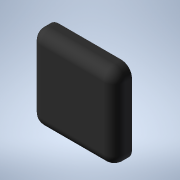
# Autodesk Inventor part: 0000-00189079(1)
Saved by Autodesk Inventor 2021 (Build 250183000, 183)
## iProperties
Created: 2025-05-05
Part Number: 0000-00189079(1)
Material: Generic
Catalog Web Link: www.cadenas.de
Description: Cap KL 2.0-Cap KL 2.0
Vendor: RITTAL
Document SubType Name: Modeling
Designer: psAdmin
Manufacturer: RITTAL
Mass: 0.993857 g
Surface Area: 6.97168 cm^2
Volume: 0.993857 cm^3
Density: 1 g/cm^3
Appearance: PSOLRGB-175-175-175
Category: PARTsolutions
Company: RITTAL
Title: 0000-00189079(1)
Author: Cadenas PARTsolutions
Comments: Cap KL 2.0
PSOL_IDENT_0: {$CADENAS_DATA/23d-libs/rittal/schaltschranksys/kleingeh/parts_kl_2_0/cap_kl_2_0.prj},188 {VTYP=3D},
PSOL_IDENT_1: {NB=0000-00189079(1)},{LINA=0000-00189079(1)},{NN=Cap KL 2.0},{DATE=27.11.2019 12:11:25},{GEOMDATE=2
PSOL_IDENT_2: 9.08.2019 12:58:38},{VERSION=},{LINEID=10},{WBVAR=DETAIL},{WBNUMERIC=DETAIL}  {NB=0000-00189079(1)},
PSOL_IDENT_3: {LINA=0000-00189079(1)},{KT=DUMMY},{BEST=0000-00189079},{DETAIL=1}
NB: 0000-00189079(1)
NN: Cap KL 2.0
NT: Cap KL 2.0
NBSYN: $BEST.($DETAIL.)
LINA: 0000-00189079(1)
CATALOG: Rittal
BEST: 0000-00189079
DETAIL: hoch
SUPPLIER: RITTAL
ARTICLENO: 0000-00189079(1)
BOMINFO: 0000-00189079(1)
CREATOR: CADENAS GmbH
Autodesk Inventor part; units mm, degrees
sketch "Sketch_4" plane through (0, 0, 0) normal (0, 1, 0) x (-1, 0, 0)
  arc A0 (7.75, -2) -> (5.75, 0) centre (5.75, -2) ccw
  line L0 (5.75, 0) -> (-5.75, 0)
  arc A1 (-5.75, 0) -> (-7.75, -2) centre (-5.75, -2) ccw
  line L1 (-7.75, -2) -> (-7.75, -3.25)
  line L2 (-7.75, -3.25) -> (7.75, -3.25)
  line L3 (7.75, -3.25) -> (7.75, -2)
  constraints: 8 end point, 4 point on circle, 2 centre point
extrude "Extrusion1" add sketch "Sketch_4" along normal mid plane 11.5
sketch "Sketch_5" plane through (0, 0, 0) normal (1, 0, 0) x (0, 1, 0)
  line L0 (5.75, 0) -> (-5.75, 0)
  arc A0 (-5.75, 0) -> (-7.75, -2) centre (-5.75, -2) ccw
  line L1 (-7.75, -2) -> (-7.75, -3.25)
  line L2 (-7.75, -3.25) -> (7.75, -3.25)
  line L3 (7.75, -3.25) -> (7.75, -2)
  arc A1 (7.75, -2) -> (5.75, 0) centre (5.75, -2) ccw
  constraints: 8 end point, 4 point on circle, 2 centre point
extrude "Extrusion2" add sketch "Sketch_5" along normal mid plane 11.5
sketch "Sketch_6" plane through (-5.75, 0, 0) normal (1, 0, 0) x (0, 0, -1)
  line L0 (3.25, 5.75) -> (0, 5.75)
  arc A0 (2, 7.75) -> (0, 5.75) centre (2, 5.75) ccw
  line L1 (2, 7.75) -> (3.25, 7.75)
  line L2 (3.25, 7.75) -> (3.25, 5.75)
  line L3 (3.25, 5.75) -> (0, 5.75)
  constraints: 8 end point, 2 point on circle, 1 centre point
revolve "Revolution1" add sketch "Sketch_6" angle 90 about axis through (-5.75, 5.75, -3.25) along (0, 0, 1)
sketch "Sketch_7" plane through (-5.75, 0, 0) normal (1, 0, 0) x (0, 0, -1)
  line L0 (0, -5.75) -> (3.25, -5.75)
  line L1 (3.25, -5.75) -> (3.25, -7.75)
  line L2 (3.25, -7.75) -> (2, -7.75)
  arc A0 (0, -5.75) -> (2, -7.75) centre (2, -5.75) ccw
  line L3 (0, -5.75) -> (3.25, -5.75)
  constraints: 8 end point, 2 point on circle, 1 centre point
revolve "Revolution2" add sketch "Sketch_7" angle 90 about axis through (-5.75, -5.75, 0) along (0, 0, -1)
sketch "Sketch_8" plane through (5.75, 0, 0) normal (1, 0, 0) x (0, 0, -1)
  line L0 (3.25, 5.75) -> (0, 5.75)
  arc A0 (2, 7.75) -> (0, 5.75) centre (2, 5.75) ccw
  line L1 (2, 7.75) -> (3.25, 7.75)
  line L2 (3.25, 7.75) -> (3.25, 5.75)
  line L3 (3.25, 5.75) -> (0, 5.75)
  constraints: 8 end point, 2 point on circle, 1 centre point
revolve "Revolution3" add sketch "Sketch_8" angle 90 about axis through (5.75, 5.75, -3.25) along (0, 0, -1)
sketch "Sketch_9" plane through (5.75, 0, 0) normal (1, 0, 0) x (0, 0, -1)
  line L0 (0, -5.75) -> (3.25, -5.75)
  line L1 (3.25, -5.75) -> (3.25, -7.75)
  line L2 (3.25, -7.75) -> (2, -7.75)
  arc A0 (0, -5.75) -> (2, -7.75) centre (2, -5.75) ccw
  line L3 (0, -5.75) -> (3.25, -5.75)
  constraints: 8 end point, 2 point on circle, 1 centre point
revolve "Revolution4" add sketch "Sketch_9" angle 90 about axis through (5.75, -5.75, 0) along (0, 0, 1)
sketch "Sketch_10" plane through (0, 0, 0) normal (0, 1, 0) x (-1, 0, 0)
  line L0 (0, 0) -> (0, -6.5)
  line L1 (0, -6.5) -> (-4.35, -6.5)
  line L2 (-4.35, -6.5) -> (-5.35, -5.2201)
  line L3 (-5.35, -5.2201) -> (-5.35, 0)
  line L4 (-5.35, 0) -> (0, 0)
  line L5 (0, 0) -> (0, -6.5)
  constraints: 12 end point
revolve "Revolution5" add sketch "Sketch_10" angle 360 about axis through (0, 0, 0) along (0, 0, 1)
ref_plane "CAP_XY" through (0, 0, 0) normal (0, 0, 1) x (1, 0, 0)
ref_plane "CAP_YZ" through (0, 0, 0) normal (1, 0, 0) x (0, 1, 0)
ref_plane "CAP_ZX" through (0, 0, 0) normal (0, 1, 0) x (0, 0, 1)
body "Solid1"
